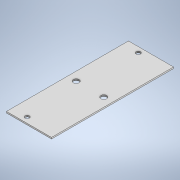
# Autodesk Inventor part: Platte4
Saved by Autodesk Inventor 2022 (Build 260153000, 153)
## iProperties
Created: 2022-04-02
Part Number: Platte4
Material: Generic
Document SubType Name: Modeling
Designer: benni
Density: 1 g/cm^3
Appearance: Default
Author: benni
Autodesk Inventor part; units mm, degrees
ref_plane "YZ Plane" through (0, 0, 0) normal (1, 0, 0) x (0, 1, 0)
ref_plane "XZ Plane" through (0, 0, 0) normal (0, 1, 0) x (-1, 0, 0)
ref_plane "XY Plane" through (0, 0, 0) normal (0, 0, 1) x (1, 0, 0)
sketch "Sketch1" plane through (0, 0, 0) normal (0, 1, 0) x (-1, 0, 0)
  line L0 (0, 0) -> (31, 0)
  line L1 (31, 0) -> (31, -84)
  line L2 (31, -84) -> (0, -84)
  line L3 (0, -84) -> (0, 0)
  line L4 (31, -42) -> (0, -42)
  circle A0 centre (20.5, -3.75) radius 1.5
  circle A1 centre (20.5, -80.25) radius 1.5
  line L5 (15.5, -84) -> (15.5, 0)
  circle A2 centre (25, -42) radius 2
  circle A3 centre (6, -42) radius 2
  dimension "d0" = 84
  dimension "d1" = 31
  dimension "d3" = 3.75
  dimension "d4" = 10.5
  dimension "d5" = 3
  dimension "d7" = 6
  dimension "d8" = 4
  constraints: 12 end point, 4 centre point, 4 midpoint, 3 coincident, 3 symmetric about line, 2 parallel, 1 horizontal, 1 perpendicular, 1 point on line, 2 other
  measures "d0" distance of L0.end L1.end
  measures "d1" distance of L1.end L2.end
  measures "d3" distance from line of L0 point (20.5, -3.75)
  measures "d4" distance from line of L1 point (20.5, -3.75)
  measures "d5" diameter of A0
  measures "d7" distance from line of L1 point (25, -42)
  measures "d8" diameter of A2
extrude "Extrusion1" add sketch "Sketch1" along normal blind 1 contours L0 L5 L4 A3 L3 | L0 L1 L4 A2 L5 | L4 A3 L5 L2 L3 | L4 A2 L1 L2 L5
body "Solid1"
